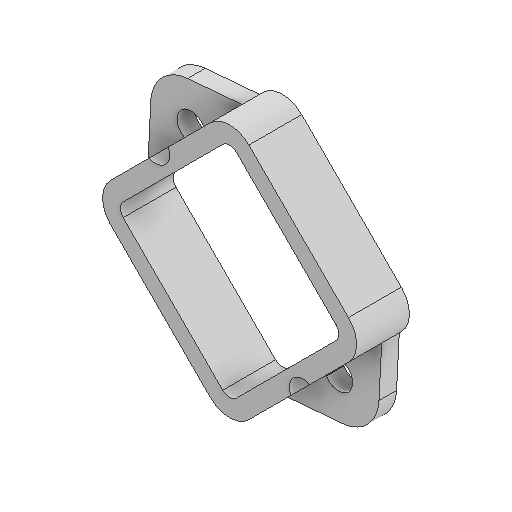
# Autodesk Inventor part: IM_Lensholder_M12
Saved by Autodesk Inventor 2022 (Build 260153000, 153)
## iProperties
Created: 2023-04-14
Part Number: IM_Lensholder_M12
Material: Generisch
Document SubType Name: Modeling
Designer: diederichbenedict
Density: 1 g/cm^3
Appearance: Vorgabe
Author: diederichbenedict
Autodesk Inventor part; units mm, degrees
ref_plane "YZ Plane" through (0, 0, 0) normal (1, 0, 0) x (0, 1, 0)
ref_plane "XZ Plane" through (0, 0, 0) normal (0, 1, 0) x (-1, 0, 0)
ref_plane "XY Plane" through (0, 0, 0) normal (0, 0, 1) x (1, 0, 0)
sketch "Skizze1" plane through (0, 0, 0) normal (0, 0, 1) x (1, 0, 0)
  circle A0 centre (0.0001, -0.0022) radius 3.9802 projected
  circle A1 centre (-8.37, 7.9978) radius 1.4 projected
  circle A2 centre (8.3745, -8.0022) radius 1.4 projected
  line L0 (-9.5383, 7.2264) -> (-3.2198, -2.3418)
  line L1 (-7.6522, 9.1998) -> (1.8915, 3.4999)
  line L2 (9.5428, -7.2307) -> (3.3215, 2.191)
  line L3 (-1.8517, -3.5253) -> (7.6567, -9.2041)
  arc A3 (12.0209, -0.7093) -> (12.0209, 0.705) centre (11.3138, -0.0022) ccw projected
  line L4 (12.0209, 0.705) -> (0.7072, 12.0187) projected
  arc A4 (0.7072, 12.0187) -> (-0.707, 12.0187) centre (0.0001, 11.3116) ccw projected
  line L5 (-0.707, 12.0187) -> (-12.0207, 0.705) projected
  arc A5 (-12.0207, 0.705) -> (-12.0207, -0.7093) centre (-11.3136, -0.0022) ccw projected
  line L6 (-12.0207, -0.7093) -> (-0.707, -12.023) projected
  arc A6 (-0.707, -12.023) -> (0.7072, -12.023) centre (0.0001, -11.3159) ccw projected
  line L7 (0.7072, -12.023) -> (12.0209, -0.7093) projected
  circle A7 centre (0.0001, -0.0022) radius 6 projected
  arc A8 (12.0916, -0.78) -> (12.0916, 0.7757) centre (11.3138, -0.0022) ccw
  line L8 (12.0916, 0.7757) -> (0.7779, 12.0894)
  arc A9 (0.7779, 12.0894) -> (-0.7777, 12.0894) centre (0.0001, 11.3116) ccw
  line L9 (-0.7777, 12.0894) -> (-12.0914, 0.7757)
  arc A10 (-12.0914, 0.7757) -> (-12.0914, -0.78) centre (-11.3136, -0.0022) ccw
  line L10 (-12.0914, -0.78) -> (-0.7777, -12.0937)
  arc A11 (-0.7777, -12.0937) -> (0.7779, -12.0937) centre (0.0001, -11.3159) ccw
  line L11 (0.7779, -12.0937) -> (12.0916, -0.78)
  circle A12 centre (8.3745, -8.0022) radius 1.6
  circle A13 centre (-8.37, 7.9978) radius 1.6
  circle A14 centre (8.3745, -8.0022) radius 4.6
  circle A15 centre (-8.37, 7.9978) radius 4.6
  line L12 (-2.1919, -13.5079) -> (-13.5056, -2.1942)
  arc A16 (-13.5056, 2.1899) -> (-13.5056, -2.1942) centre (-11.3136, -0.0022) ccw
  line L13 (-13.5056, 2.1899) -> (-2.1919, 13.5036)
  arc A17 (2.1922, 13.5036) -> (-2.1919, 13.5036) centre (0.0001, 11.3116) ccw
  line L14 (2.1922, 13.5036) -> (13.5059, 2.1899)
  arc A18 (13.5059, -2.1942) -> (13.5059, 2.1899) centre (11.3138, -0.0022) ccw
  line L15 (13.5059, -2.1942) -> (2.1922, -13.5079)
  arc A19 (-2.1919, -13.5079) -> (2.1922, -13.5079) centre (0.0001, -11.3159) ccw
  line L16 (-2.1919, -13.5079) -> (8.3745, -12.6022)
  line L17 (13.5059, 2.1899) -> (12.9684, -8.2389)
  line L18 (2.1922, 13.5036) -> (-8.756, 12.5816)
  line L19 (-13.4843, -2.2153) -> (-12.9668, 7.8266)
  point P0 (0, 0)
  point P1 (13.2677, -2.4324)
  point P2 (-2.595, 13.1004)
  point P3 (-13.2438, 2.4517)
  point P4 (2.6032, -13.0969)
  point P5 (-6.9281, 8.7674)
  point P6 (-6.9536, 8.7419)
  point P7 (-6.9872, 8.8026)
  point P8 (6.93, -8.7701)
  point P9 (6.9566, -8.7434)
  point P10 (9.1158, -6.5842)
  point P11 (9.1159, -6.5842)
  point P12 (9.116, -6.5843)
  point P13 (6.9917, -8.8069)
  dimension "d15" = 0.1
  dimension "d16" = 3.2
  dimension "d17" = 3.2
  dimension "d18" = 3
  dimension "d19" = 3
  dimension "d20" = 2
  constraints: 32 end point, 29 point on circle, 12 centre point, 7 tangent, 2 coincident, 2 parallel, 14 other
  measures "d15" distance between parallel lines of L7 L11
  measures "d16" diameter of A12
  measures "d17" diameter of A13
  measures "d18" radial gap between concentric circles of A12 A14
  measures "d19" radial gap between concentric circles of A13 A15
  measures "d20" distance between parallel lines of L10 L12
extrude "Extrusion4" add sketch "Skizze1" along normal blind 2 contours L11 A14 L15 L2 | L2 A12 L15 L3 L11 | L11 A8 L8 A9 L9 A15 L13 L18 L14 L17 L15 A14 | L3 L15 A14 L11 | A14 L15 L16 L12 L19 L13 A15 L9 A10 L10 A11 L11 | L9 L0 A13 L13 L1 | L1 L13 A15 L9 | L15 A14 L3 A12 | L15 L17 A14 | L9 A15 L13 L0 | A14 L16 L15 | L1 A13 L13 A15 | L17 A18 L15 | L13 L19 A15 | L15 A19 L16 | A15 L18 L13 | L19 L12 A16 L13 | L13 A17 L18
sketch "Skizze5" plane through (0, 0, 2) normal (0, 0, 1) x (1, 0, 0)
  line L0 (12.9684, -8.2389) -> (13.2677, -2.4324) projected
  line L1 (13.2677, -2.4324) -> (13.5059, -2.1942) projected
  arc A0 (13.5059, -2.1942) -> (13.5059, 2.1899) centre (11.3138, -0.0022) ccw projected
  line L2 (13.5059, 2.1899) -> (2.1922, 13.5036) projected
  arc A1 (2.1922, 13.5036) -> (-2.1919, 13.5036) centre (0.0001, 11.3116) ccw projected
  line L3 (-2.1919, 13.5036) -> (-2.595, 13.1004) projected
  line L4 (-2.595, 13.1004) -> (-8.756, 12.5816) projected
  arc A2 (-8.756, 12.5816) -> (-12.9668, 7.8266) centre (-8.37, 7.9978) ccw projected
  line L5 (-12.9668, 7.8266) -> (-13.2438, 2.4517) projected
  line L6 (-13.2438, 2.4517) -> (-13.5056, 2.1899) projected
  arc A3 (-13.5056, 2.1899) -> (-13.5056, -2.1942) centre (-11.3136, -0.0022) ccw projected
  line L7 (-13.5056, -2.1942) -> (-2.1919, -13.5079) projected
  arc A4 (-2.1919, -13.5079) -> (2.1922, -13.5079) centre (0.0001, -11.3159) ccw projected
  line L8 (2.1922, -13.5079) -> (2.6032, -13.0969) projected
  line L9 (2.6032, -13.0969) -> (8.3745, -12.6022) projected
  arc A5 (8.3745, -12.6022) -> (12.9684, -8.2389) centre (8.3745, -8.0022) ccw projected
  line L10 (-12.0914, 0.7757) -> (-0.7777, 12.0894) projected
  arc A6 (0.7779, 12.0894) -> (-0.7777, 12.0894) centre (0.0001, 11.3116) ccw projected
  line L11 (0.7779, 12.0894) -> (12.0916, 0.7757) projected
  arc A7 (12.0916, -0.78) -> (12.0916, 0.7757) centre (11.3138, -0.0022) ccw projected
  line L12 (12.0916, -0.78) -> (0.7779, -12.0937) projected
  arc A8 (-0.7777, -12.0937) -> (0.7779, -12.0937) centre (0.0001, -11.3159) ccw projected
  line L13 (-0.7777, -12.0937) -> (-12.0914, -0.78) projected
  arc A9 (-12.0914, 0.7757) -> (-12.0914, -0.78) centre (-11.3136, -0.0022) ccw projected
  line L14 (-6.9281, 8.7674) -> (-6.9536, 8.7419) projected
  arc A10 (-6.9872, 8.8026) -> (-6.9536, 8.7419) centre (-8.37, 7.9978) ccw projected
  line L15 (-6.9872, 8.8026) -> (-6.9281, 8.7674) projected
  line L16 (6.93, -8.7701) -> (6.9566, -8.7434) projected
  arc A11 (9.1158, -6.5842) -> (6.9566, -8.7434) centre (8.3745, -8.0022) ccw projected
  line L17 (9.1158, -6.5842) -> (9.1159, -6.5842) projected
  line L18 (9.1159, -6.5842) -> (9.116, -6.5843) projected
  arc A12 (6.9917, -8.8069) -> (9.116, -6.5843) centre (8.3745, -8.0022) ccw projected
  line L19 (6.9917, -8.8069) -> (6.93, -8.7701) projected
  line L20 (12.9684, -8.2389) -> (13.2677, -2.4324) projected
  line L21 (2.6032, -13.0969) -> (13.2677, -2.4324)
  line L22 (-2.595, 13.1004) -> (-8.756, 12.5816) projected
  line L23 (-2.595, 13.1004) -> (-13.2438, 2.4517)
  point P0 (0, 0)
  point P1 (-9.1141, 6.5814)
  constraints: 4 end point, 1 parallel
extrude "Extrusion5" add sketch "Skizze5" along normal blind 4 contours L21 A11 L16 L8 A4 L7 A3 L6 L23 A10 L14 L3 A1 L2 A0 L1
